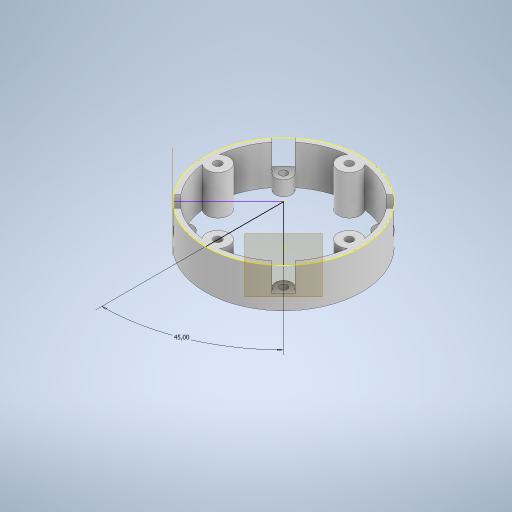
# Autodesk Inventor part: cylinder
Saved by Autodesk Inventor 2024 (Build 280153000, 153)
## iProperties
Created: 2024-05-02
Part Number: cylinder
Material: Generic
Document SubType Name: Modeling
Designer: david
Density: 1 g/cm^3
Appearance: Default
Author: david
Autodesk Inventor part; units mm, degrees
ref_plane "YZ Plane" through (0, 0, 0) normal (1, 0, 0) x (0, 1, 0)
ref_plane "XZ Plane" through (0, 0, 0) normal (0, 1, 0) x (-1, 0, 0)
ref_plane "XY Plane" through (0, 0, 0) normal (0, 0, 1) x (1, 0, 0)
sketch "Sketch1" plane through (0, 0, 0) normal (0, 1, 0) x (-1, 0, 0)
  circle A0 centre (0, 0) radius 31.5
  circle A1 centre (0, 0) radius 29.5
  dimension "d0" = 63
  dimension "d1" = 59
  constraints: 2 centre point, 2 coincident
  measures "d0" diameter of A0
  measures "d1" diameter of A1
extrude "Walls" add sketch "Sketch1" along normal blind 15.9
sketch "Sketch2" plane through (0, 0, 0) normal (0, -1, 0) x (1, 0, 0)
  circle A0 centre (0, 0) radius 31.5 projected
  line L0 (0, -31.5) -> (0, -26.5)
  circle A1 centre (0, -26.5) radius 2.75
  circle A2 centre (0, -26.5) radius 4.5
  circle A3 centre (26.5, 0) radius 4.5
  circle A4 centre (26.5, 0) radius 2.75
  circle A5 centre (0, 26.5) radius 4.5
  circle A6 centre (0, 26.5) radius 2.75
  circle A7 centre (-26.5, 0) radius 4.5
  circle A8 centre (-26.5, 0) radius 2.75
  dimension "d4" = 5
  dimension "d5" = 5.5
  dimension "d6" = 9
  dimension "d9" = 360
  constraints: 8 centre point, 5 coincident, 2 end point, 1 vertical, 1 vertical alignment, 18 other
  measures "d4" distance of L0.start L0.end
  measures "d5" diameter of A1
  measures "d6" diameter of A2
extrude "Pillar holes" add sketch "Sketch2" against normal blind 15.9 contours A2 | A3 | A5 | A7
sketch "Sketch4" plane through (0, 15.9, 0) normal (0, 1, 0) x (1, 0, 0)
  point P0 (0, 0)
sketch "Sketch5" plane through (0, 0, 0) normal (0, -1, 0) x (1, 0, 0)
  point P0 (0, 0)
sketch "Sketch6" plane through (0, 15.9, 0) normal (0, 1, 0) x (1, 0, 0)
  circle A0 centre (0, 26.5) radius 2.75 projected
  circle A1 centre (0, 26.5) radius 2.75
  circle A2 centre (0, 26.5) radius 1.55
  circle A3 centre (-26.5, 0) radius 1.55
  circle A4 centre (-26.5, 0) radius 2.75
  circle A5 centre (0, -26.5) radius 1.55
  circle A6 centre (0, -26.5) radius 2.75
  circle A7 centre (26.5, 0) radius 1.55
  circle A8 centre (26.5, 0) radius 2.75
  point P0 (0, 0)
  dimension "d20" = 3.1
  dimension "d23" = 360
  constraints: 8 centre point, 5 coincident, 17 other
  measures "d20" diameter of A2
extrude "Extrusion4" add sketch "Sketch6" against normal blind 8
sketch "Sketch7" plane through (0, 15.9, 0) normal (0, 1, 0) x (1, 0, 0)
  line L0 (0, 0) -> (22.2739, -22.2739)
  circle A0 centre (0, 0) radius 31.5 projected
  line L1 (0, 0) -> (0, -31.5)
  line L2 (0, 0) -> (-22.2739, -22.2739)
  dimension "d27" = 45
  constraints: 6 end point, 3 point on circle, 1 vertical
  measures "d27" angle of L0 L1
ref_plane "Work Plane1" through (22.2739, 15.9, 22.2739) normal (0.7071, 0, 0.7071) x (0, 1, 0)
ref_plane "Work Plane2" through (-22.2739, 15.9, 22.2739) normal (-0.7071, 0, 0.7071) x (0, -1, 0)
sketch "Sketch17" plane through (0, 15.9, 0) normal (0, 1, 0) x (1, 0, 0)
  line L0 (0, 0) -> (-22.2739, -22.2739)
  line L1 (0, 0) -> (0, -14.1086)
  line L2 (-22.2739, -22.2739) -> (-19.9135, -19.9135)
  circle A0 centre (-19.9135, -19.9135) radius 1.55
  circle A1 centre (-19.9135, -19.9135) radius 3.338
  circle A2 centre (19.9135, -19.9135) radius 1.55
  circle A3 centre (19.9135, -19.9135) radius 3.338
  circle A4 centre (19.9135, 19.9135) radius 1.55
  circle A5 centre (19.9135, 19.9135) radius 3.338
  circle A6 centre (-19.9135, 19.9135) radius 1.55
  circle A7 centre (-19.9135, 19.9135) radius 3.338
  point P0 (22.2739, -22.2739)
  point P1 (22.2739, 22.2739)
  point P2 (-22.2739, 22.2739)
  dimension "d86" = 31.5
  dimension "d87" = 45
  dimension "d88" = 3.338
  dimension "d89" = 3.1
  dimension "d92" = 360
  constraints: 6 end point, 5 coincident, 4 centre point, 1 point on line, 1 vertical, 33 other
  measures "d86" distance of L0.start L0.end
  measures "d87" angle of L1 L0
  measures "d88" distance of L0.end L2.end
  measures "d89" diameter of A0
extrude "Extrusion13" add sketch "Sketch17" against normal blind 15.9 contours A1 L0 A0 | L0 A0 A1 | A0 L0 | L0 A0 | A2 | A3 | A4 | A5 | A6 | A7
sketch "Sketch18" plane through (0, 15.9, 0) normal (0, 1, 0) x (1, 0, 0)
  circle A0 centre (0, 0) radius 31.5 projected
  line L0 (0, 0) -> (-22.2739, -22.2739)
  line L1 (0, 0) -> (0, -10.409)
  line L2 (-22.2739, -22.2739) -> (-19.9135, -19.9135)
  circle A1 centre (-19.9135, -19.9135) radius 1.55
  circle A2 centre (19.9135, -19.9135) radius 1.55
  circle A3 centre (19.9135, 19.9135) radius 1.55
  circle A4 centre (-19.9135, 19.9135) radius 1.55
  dimension "d96" = 45
  dimension "d97" = 3.338
  dimension "d98" = 3.1
  dimension "d101" = 360
  constraints: 6 end point, 4 centre point, 1 coincident, 1 point on line, 1 vertical, 11 other
  measures "d96" angle of L0 L1
  measures "d97" distance of L0.end L2.end
  measures "d98" diameter of A1
extrude "Extrusion14" cut sketch "Sketch18" against normal blind 15.9 contours A1 L0 | L0 A1 | A2 | A3 | A4
sketch "Sketch19" plane through (0, 15.9, 0) normal (0, 1, 0) x (1, 0, 0)
  arc A0 (22.9523, -18.5322) -> (18.5322, -22.9523) centre (19.9135, -19.9135) ccw projected
  circle A1 centre (19.9135, -19.9135) radius 3.338
  circle A2 centre (19.9135, -19.9135) radius 1.55 projected
  line L0 (19.9135, -19.9135) -> (17.5532, -22.2739)
  line L1 (19.9135, -19.9135) -> (22.2739, -17.5532)
  line L2 (17.5532, -22.2739) -> (19.7881, -24.5088)
  circle A3 centre (0, 0) radius 31.5 projected
  line L3 (22.2739, -17.5532) -> (24.5088, -19.7881)
  line L4 (17.5532, -17.5532) -> (19.9135, -15.1929)
  line L5 (19.9135, -15.1929) -> (22.2739, -17.5532)
  line L6 (17.5532, -17.5532) -> (15.1929, -19.9135)
  line L7 (15.1929, -19.9135) -> (17.5532, -22.2739)
  arc A4 (19.7881, -24.5088) -> (24.5088, -19.7881) centre (0, 0) ccw
  line L8 (19.9135, 15.1929) -> (22.2739, 17.5532)
  line L9 (22.2739, 17.5532) -> (24.5088, 19.7881)
  arc A5 (24.5088, 19.7881) -> (19.7881, 24.5088) centre (0, 0) ccw
  circle A6 centre (19.9135, 19.9135) radius 3.338
  line L10 (17.5532, 17.5532) -> (15.1929, 19.9135)
  line L11 (17.5532, 17.5532) -> (19.9135, 15.1929)
  line L12 (15.1929, 19.9135) -> (17.5532, 22.2739)
  line L13 (17.5532, 22.2739) -> (19.7881, 24.5088)
  line L14 (-15.1929, 19.9135) -> (-17.5532, 22.2739)
  line L15 (-17.5532, 22.2739) -> (-19.7881, 24.5088)
  arc A7 (-19.7881, 24.5088) -> (-24.5088, 19.7881) centre (0, 0) ccw
  circle A8 centre (-19.9135, 19.9135) radius 3.338
  line L16 (-17.5532, 17.5532) -> (-19.9135, 15.1929)
  line L17 (-17.5532, 17.5532) -> (-15.1929, 19.9135)
  line L18 (-19.9135, 15.1929) -> (-22.2739, 17.5532)
  line L19 (-22.2739, 17.5532) -> (-24.5088, 19.7881)
  line L20 (-19.9135, -15.1929) -> (-22.2739, -17.5532)
  line L21 (-22.2739, -17.5532) -> (-24.5088, -19.7881)
  arc A9 (-24.5088, -19.7881) -> (-19.7881, -24.5088) centre (0, 0) ccw
  circle A10 centre (-19.9135, -19.9135) radius 3.338
  line L22 (-17.5532, -17.5532) -> (-15.1929, -19.9135)
  line L23 (-17.5532, -17.5532) -> (-19.9135, -15.1929)
  line L24 (-15.1929, -19.9135) -> (-17.5532, -22.2739)
  line L25 (-17.5532, -22.2739) -> (-19.7881, -24.5088)
  line L26 (19.9135, -15.1929) -> (24.5088, -19.7881)
  line L27 (15.1929, -19.9135) -> (19.7881, -24.5088)
  line L28 (19.9135, -15.1929) -> (15.1929, -19.9135)
  arc A11 (19.7881, -24.5088) -> (24.5088, -19.7881) centre (0, 0) ccw
  point P0 (19.7881, 24.5088)
  point P1 (-24.5088, 19.7881)
  point P2 (-19.7881, -24.5088)
  dimension "d107" = 360
  constraints: 58 end point, 25 point on circle, 9 centre point, 6 tangent, 5 point on line, 3 parallel, 3 perpendicular, 2 collinear, 2 concentric, 1 coincident, 69 other
extrude "Extrusion15" cut sketch "Sketch19" against normal blind 10 contours A1 A0 L0 A2 L1 | A0 L3 A3 A1 | L1 A2 L0 A0 | A3 L2 A0 A1 | L9 A6 A3 | A3 A10 L25 | A6 L13 A3 | A6 | A3 L21 A10 | A10 | L15 A8 A3 | A3 A8 L19 | A8
body "Solid1"
